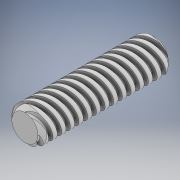
# Autodesk Inventor part: ACME 8mm Lead Screw 2mm-pitch
Saved by Autodesk Inventor 2020.3 (Build 243373000, 373)
## iProperties
Created: 2021-01-08
Part Number: ACME 8mm Lead Screw 2mm-pitch
Material: Generic
Document SubType Name: Modeling
Designer: Johnson Ebenezer R
Density: 1 g/cm^3
Appearance: Default
Author: Johnson Ebenezer R
Autodesk Inventor part; units mm, degrees
ref_plane "YZ Plane" through (0, 0, 0) normal (1, 0, 0) x (0, 1, 0)
ref_plane "XZ Plane" through (0, 0, 0) normal (0, 1, 0) x (-1, 0, 0)
ref_plane "XY Plane" through (0, 0, 0) normal (0, 0, 1) x (1, 0, 0)
sketch "Sketch1" plane through (0, 0, 0) normal (0, 0, 1) x (1, 0, 0)
  circle A0 centre (0, 0) radius 4
  dimension "dia" = 8
  constraints: 1 centre point, 1 coincident
  measures "dia" diameter of A0
extrude "Extrusion1" add sketch "Sketch1" against normal blind 30
chamfer "Chamfer1" distance 1 angle 45 2 edges at (-4, 0, 0) (-4, 0, -30)
sketch "Sketch2" plane through (0, 0, 0) normal (1, 0, 0) x (0, 1, 0)
  line L0 (4, 2.3379) -> (4, -4.3379)
  line L1 (4, -1) -> (-4, -1) projected
  line L2 (4, -0.2586) -> (3, -0.1293)
  line L3 (3, -0.1293) -> (3, 0.6121)
  line L4 (3, 0.6121) -> (4, 0.7414)
  line L5 (0, 0) -> (0, -30)
  line L6 (3, -30) -> (-3, -30) projected
  dimension "d10" = 0.7414
  dimension "d11" = 1
  dimension "d12" = 0.7414
  dimension "d13" = 1
  constraints: 10 end point, 3 midpoint, 3 point on line, 2 vertical, 1 equal length
  measures "d10" distance from line of L2.start L1
  measures "d11" distance of L2.start L4.end
  measures "d12" distance of L2.end L3.end
  measures "d13" distance between parallel lines of L3 L0
coil "Coil1" sketch "Sketch2" operation cut axis through (0, 0, 0) along (0, 0, -1) pitch 8 turns 3.75 hand right
pattern_circular "Circular Pattern7" count 4 over 360 about axis through (0, 0, -29.5) along (0, 0, -1) of "Coil1"
equation "\"d10\" = 0.3707 * p"
equation "\"d11\" = 0.5 * p"
equation "\"d12\" = d10"
equation "\"d13\" = 0.5 * p"
equation "\"d14\" = 4 * p"
equation "\"p\" = 2"
body "Solid1"
